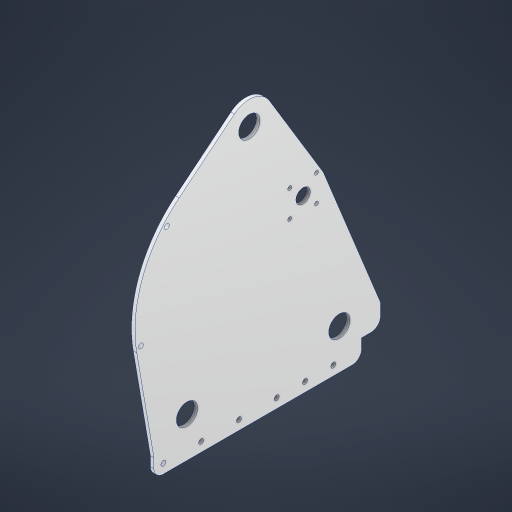
# Autodesk Inventor part: CORL_001_MainPlate
Saved by Autodesk Inventor 2024.2 (Build 282272000, 272)
## iProperties
Created: 2024-08-01
Part Number: CORL_001_MainPlate
Material: Aluminum 6061
Document SubType Name: Modeling
Designer: Bryan
Density: 2.7 g/cm^3
Appearance: Aluminum - Flat
Mass: 357.689 g
Surface Area: 1779.61 cm^2
Volume: 357.689 cm^3
Author: Bryan
Autodesk Inventor part; units mm, degrees
ref_plane "YZ Plane" through (0, 0, 0) normal (1, 0, 0) x (0, 1, 0)
ref_plane "XZ Plane" through (0, 0, 0) normal (0, 1, 0) x (-1, 0, 0)
ref_plane "XY Plane" through (0, 0, 0) normal (0, 0, 1) x (1, 0, 0)
sketch "Sketch1" plane through (0, 0, 0) normal (1, 0, 0) x (0, 1, 0)
  line L0 (0, 0) -> (0, -205.0034) construction
  circle A0 centre (0, 0) radius 25.4 construction
  circle A1 centre (0, -205.0034) radius 25.4 construction
  circle A2 centre (0, 0) radius 14.2875
  circle A3 centre (0, -205.0034) radius 14.2875
  line L1 (0, -266.7) -> (406.4, -266.7) construction
  line L2 (0, 0) -> (0, 69.85) construction
  line L3 (0, 69.85) -> (406.4, 69.85) construction
  line L4 (-25.4, 0) -> (-25.4, -205.0034) construction
  arc A4 (-25.4, 0) -> (-25.4, 0) centre (0, 0) ccw construction
  arc A5 (-25.4, -205.0034) -> (0, -230.4034) centre (0, -205.0034) ccw construction
  line L5 (-53.975, 44.45) -> (-28.575, 44.45)
  line L6 (-28.575, 44.45) -> (-28.575, -234.95) construction
  line L7 (-28.575, -234.95) -> (-53.975, -234.95)
  line L8 (-53.975, -234.95) -> (-53.975, 44.45)
  line L9 (-28.575, -234.95) -> (-28.575, -260.35)
  circle A6 centre (-41.275, 44.45) radius 3.2512 construction
  circle A7 centre (-41.275, 31.75) radius 3.2512
  circle A8 centre (-41.275, 19.05) radius 3.2512 construction
  circle A9 centre (-41.275, 6.35) radius 3.2512 construction
  circle A10 centre (-41.275, -6.35) radius 3.2512 construction
  circle A11 centre (-41.275, -19.05) radius 3.2512
  circle A12 centre (-41.275, -31.75) radius 3.2512 construction
  circle A13 centre (-41.275, -44.45) radius 3.2512 construction
  circle A14 centre (-41.275, -57.15) radius 3.2512 construction
  circle A15 centre (-41.275, -69.85) radius 3.2512
  circle A16 centre (-41.275, -82.55) radius 3.2512 construction
  circle A17 centre (-41.275, -95.25) radius 3.2512 construction
  circle A18 centre (-41.275, -107.95) radius 3.2512 construction
  circle A19 centre (-41.275, -120.65) radius 3.2512
  circle A20 centre (-41.275, -133.35) radius 3.2512 construction
  circle A21 centre (-41.275, -146.05) radius 3.2512 construction
  circle A22 centre (-41.275, -158.75) radius 3.2512
  circle A23 centre (-41.275, -171.45) radius 3.2512 construction
  circle A24 centre (-41.275, -184.15) radius 3.2512 construction
  circle A25 centre (-41.275, -196.85) radius 3.2512
  circle A26 centre (-41.275, -209.55) radius 3.2512 construction
  circle A27 centre (-41.275, -222.25) radius 3.2512 construction
  circle A28 centre (-41.275, -234.95) radius 3.2512 construction
  line L10 (0, -205.0034) -> (146.8616, -164.2919) construction
  circle A29 centre (176.2339, -156.1495) radius 30.48 construction
  circle A30 centre (176.2339, -156.1495) radius 9.525
  circle A31 centre (176.2339, -156.1495) radius 30 construction
  circle A32 centre (194.1944, -174.1101) radius 2.4892
  circle A33 centre (158.2734, -174.1101) radius 2.4892
  circle A34 centre (194.1944, -138.189) radius 2.4892
  circle A35 centre (158.2734, -138.189) radius 2.4892
  line L11 (194.1944, -138.189) -> (158.2734, -138.189) construction
  line L12 (158.2734, -138.189) -> (158.2734, -174.1101) construction
  line L13 (158.2734, -174.1101) -> (194.1944, -174.1101) construction
  line L14 (194.1944, -174.1101) -> (194.1944, -138.189) construction
  circle A36 centre (176.2339, -156.1495) radius 25.4 construction
  line L15 (0, 0) -> (249.8384, -215.9) construction
  circle A37 centre (293.0267, -83.8953) radius 25.4 construction
  arc A38 (293.0267, -83.8953) -> (0, 0) centre (132.5272, -90.7978) ccw construction
  line L16 (0, -205.0034) -> (59.0925, -345.4806) construction
  line L17 (59.0925, -345.4806) -> (281.6851, -514.35) construction
  circle A39 centre (281.6851, -514.35) radius 50.8 construction
  line L18 (294.3851, -565.15) -> (268.9851, -565.15) construction
  circle A40 centre (59.0925, -345.4806) radius 50.8 construction
  circle A41 centre (0, -205.0034) radius 152.4 construction
  line L19 (0, -205.0034) -> (152.0099, -215.9) construction
  line L20 (152.0099, -215.9) -> (403.3467, -93.8582) construction
  circle A42 centre (403.3467, -93.8582) radius 50.8 construction
  circle A43 centre (152.0099, -215.9) radius 50.8 construction
  line L21 (293.0267, -83.8953) -> (232.107, 27.0652) construction
  circle A44 centre (232.107, 27.0652) radius 6.35 construction
  circle A45 centre (232.107, 27.0652) radius 3.2512
  circle A46 centre (293.0267, -83.8953) radius 14.2875
  circle A47 centre (403.3467, -93.8582) radius 25.4 construction
  circle A48 centre (152.0099, -215.9) radius 25.4 construction
  line L22 (392.252, -71.0094) -> (140.9152, -193.0512) construction
  line L23 (163.1047, -238.7488) -> (414.4414, -116.707) construction
  circle A49 centre (293.0267, -83.8953) radius 31.75 construction
  circle A50 centre (59.0925, -345.4806) radius 25.4 construction
  line L24 (0, -205.0034) -> (80.5364, -331.8675) construction
  circle A51 centre (110.4127, 61.907) radius 6.35 construction
  circle A52 centre (110.4127, 61.907) radius 3.2512
  line L25 (232.107, 27.0652) -> (110.4127, 61.907) construction
  line L26 (110.4127, 61.907) -> (0, 0) construction
  line L27 (-28.575, 44.45) -> (105.239, 67.5154)
  line L28 (257.1863, 10.5325) -> (317.6639, -63.8686)
  arc A53 (257.1863, 10.5325) -> (105.239, 67.5154) centre (132.5272, -90.7978) ccw
  line L29 (-28.575, -260.35) -> (0, -260.35)
  arc A54 (309.4803, -111.0493) -> (317.6639, -63.8686) centre (293.0267, -83.8953) ccw
  line L30 (309.4803, -111.0493) -> (192.0294, -182.2174)
  line L31 (187.6679, -184.4036) -> (0, -260.35)
  arc A55 (187.6679, -184.4036) -> (192.0294, -182.2174) centre (176.2339, -156.1495) ccw
  point P0 (-41.275, 44.45)
  point P1 (281.6851, -565.15)
  dimension "d165" = 50.8
  dimension "d0" = 205.0034
  dimension "d1" = 50.8
  dimension "d3" = 28.575
  dimension "d4" = 28.575
  dimension "d15" = 69.85
  dimension "d19" = 25.4
  dimension "d21" = 3.175
  dimension "d22" = 44.45
  dimension "d23" = 6.5024
  dimension "d27" = 12.7
  dimension "d68" = 60.96
  dimension "d73" = 152.4
  dimension "d74" = 19.05
  dimension "d93" = 60
  dimension "d130" = 4.9784
  dimension "d132" = 50.8
  dimension "d133" = 279.4
  dimension "d139" = 25.4
  dimension "d144" = 6.35
  dimension "d145" = 406.4
  dimension "d147" = 330.2
  dimension "d148" = 50.8
  dimension "d149" = 304.8
  dimension "d151" = 50.8
  dimension "d152" = 279.4
  dimension "d153" = 101.6
  dimension "d154" = 304.8
  dimension "d155" = 150
  dimension "d156" = 150
  dimension "d157" = 12.7
  dimension "d158" = 6.5024
  dimension "d161" = 317.0675
  dimension "d162" = 50.8
  dimension "d163" = 50.8
  dimension "d164" = 63.5
  dimension "d166" = 12.7
  dimension "d167" = 6.5024
  dimension "d168" = 9.594
  dimension "d170" = 19.594
  constraints: 65 end point, 54 centre point, 29 point on circle, 25 coincident, 20 tangent, 11 equal radius, 8 equal length, 7 vertical, 6 horizontal, 4 vertical alignment, 3 midpoint, 3 parallel, 1 concentric, 1 perpendicular, 1 point on line, 52 other
  measures "d0" distance of L0.start L0.end
  measures "d1" diameter of A0
  measures "d3" diameter of A2
  measures "d4" diameter of A3
  measures "d15" distance of L2.start L2.end
  measures "d19" distance of L5.start L5.end
  measures "d21" distance between parallel lines of L4 L6
  measures "d22" distance from line of L5 L0.start
  measures "d23" diameter of A6
  measures "d27" distance of A6.centre A7.centre
  measures "d68" diameter of A29
  measures "d73" distance of L0.end L10.end
  measures "d74" diameter of A30
  measures "d93" diameter of A31
  measures "d130" diameter of A32
  measures "d132" diameter of A36
  measures "d133" distance between parallel lines of L5 L7
  measures "d139" distance of L6.end L9.end
  measures "d144" vertical distance of L9.end L1.start
  measures "d145" distance of L2.end L3.end
  measures "d147" distance of L0.start L15.end
  measures "d148" diameter of A37
  measures "d149" distance of L0.start L21.start
  measures "d151" vertical distance of L1.end L15.end
  measures "d152" distance of L16.end L17.end
  measures "d153" diameter of A39
  measures "d154" distance from line of L9.end L18
  measures "d155" angle of L17 L16
  measures "d156" angle of L19 L20
  measures "d157" diameter of A44
  measures "d158" diameter of A45
  measures "d161" distance of L0.end A46.centre
  measures "d162" diameter of A47
  measures "d163" diameter of A48
  measures "d164" diameter of A49
  measures "d166" diameter of A51
  measures "d167" diameter of A52
  measures "d168" angle of L16 L24
  measures "d170" angle of L19 L10
extrude "Extrusion1" add sketch "Sketch1" along normal blind 4.7625
fillet "Fillet2" radius 12.7 3 edges at (2.3813, -53.975, 44.45) (2.3813, -53.975, -234.95) (2.3813, -28.575, -260.35)
body "Solid1"
